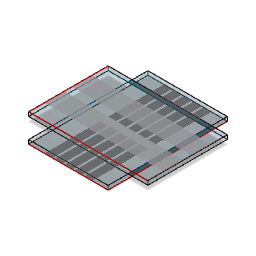
Assembly (Autodesk Fusion 360 archive; units mm, degrees)
design "TCA Test Structure"
Autodesk Fusion 360 part; units mm, degrees
sketch "Sketch1" plane through (0, 0, 0) normal (0, 1, 0) x (1, 0, 0)
  line L0 (10, -15) -> (-10, -15)
  line L1 (-10, -15) -> (-10, 15)
  line L2 (-10, 15) -> (10, 15)
  line L3 (10, 15) -> (10, -15)
  line L4 (10, -15) -> (-10, 15) construction
  line L5 (-10, -15) -> (10, 15) construction
  dimension "d1" = 20
  dimension "d2" = 30
  constraint perpendicular L0 L1
  constraint parallel L0 L2
  constraint parallel L1 L3
  constraint horizontal L0
  constraint coincident L4 origin
  constraint coincident L5 origin
  measures "d1" distance of L1.end L2.end
  measures "d2" distance of L0.end L1.end
extrude "Extrude1" add sketch "Sketch1" along normal blind 1
sketch "Sketch2" plane through (0, 1, 0) normal (0, 1, 0) x (-1, 0, 0)
  line L0 (-10, -15) -> (10, -15)
  line L1 (10, -15) -> (10, 15)
  line L2 (10, 15) -> (-10, 15)
  line L3 (-10, 15) -> (-10, -15)
  line L4 (-10, 10) -> (10, 10)
  line L5 (10, 10) -> (10, -10)
  line L6 (10, -10) -> (-10, -10)
  line L7 (-10, -10) -> (-10, 10)
  line L8 (-10, 10) -> (10, -10) construction
  line L9 (10, 10) -> (-10, -10) construction
  dimension "d5" = 20
  constraint perpendicular L4 L5
  constraint parallel L4 L6
  constraint parallel L5 L7
  constraint horizontal L4
  constraint coincident L3 L4.start
  constraint coincident L8 origin
  constraint coincident L9 origin
  measures "d5" distance of L4.end L5.end
extrude "Extrude2" add sketch "Sketch2" along normal blind 0.04 contours L1 L3 L4 L5 L6 L7
sketch "Sketch3" plane through (0, 1.04, 0) normal (0, 1, 0) x (-1, 0, 0)
  line L0 (-10, -10) -> (10, -10)
  line L1 (10, -10) -> (10, 10)
  line L2 (10, 10) -> (-10, 10)
  line L3 (-10, 10) -> (-10, -10)
  line L4 (-15, 10) -> (15, 10)
  line L5 (15, 10) -> (15, -10)
  line L6 (15, -10) -> (-15, -10)
  line L7 (-15, -10) -> (-15, 10)
  line L8 (-15, 10) -> (15, -10) construction
  line L9 (15, 10) -> (-15, -10) construction
  dimension "d8" = 30
  dimension "d9" = 20
  constraint perpendicular L4 L5
  constraint parallel L4 L6
  constraint parallel L5 L7
  constraint horizontal L4
  constraint coincident L8 origin
  constraint coincident L9 origin
  measures "d8" distance of L5.end L6.end
  measures "d9" distance of L4.end L5.end
extrude "Extrude3" add sketch "Sketch3" along normal blind 1

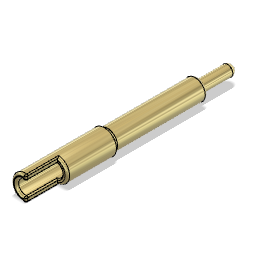
design "Pin-0955-0-15-20-71-14-11-0"
Autodesk Fusion 360 part; units mm, degrees
sketch "Sketch1" plane through (0, 0, 0) normal (0, 1, 0) x (1, 0, 0)
  line L0 (0, 0) -> (0, -7.65)
  line L1 (-0.445, 0) -> (0.445, 0)
  line L2 (0.445, 0) -> (0.445, -4.09)
  line L3 (0.445, -4.09) -> (-0.445, -4.09)
  line L4 (-0.445, -4.09) -> (-0.445, 0)
  line L5 (-0.535, -4.09) -> (0.535, -4.09)
  line L6 (0.535, -4.09) -> (0.535, -7.65)
  line L7 (0.535, -7.65) -> (-0.535, -7.65)
  line L8 (-0.535, -7.65) -> (-0.535, -4.09)
  line L9 (-0.305, -7.65) -> (0.305, -7.65)
  line L10 (0.305, -7.65) -> (0.305, -5.11)
  line L11 (0.305, -5.11) -> (-0.305, -5.11)
  line L12 (-0.305, -5.11) -> (-0.305, -7.65)
  line L13 (-0.24, 0) -> (0.24, 0)
  line L14 (0.24, 0) -> (0.24, 1.55)
  line L15 (0.24, 1.55) -> (-0.24, 1.55)
  line L16 (-0.24, 1.55) -> (-0.24, 0)
  circle A0 centre (-0.000074, 1.309926) radius 0.240074
  line L17 (0, 0) -> (0, 1.55)
  dimension "d1" = 7.65
  dimension "d2" = 4.09
  dimension "d3" = 0.89
  dimension "d4" = 3.56
  dimension "d5" = 1.07
  dimension "d6" = 0.61
  dimension "d7" = 2.54
  dimension "d8" = 0.48
  dimension "d9" = 1.55
  constraint coincident L0.start L17.start
  constraint vertical L0
  constraint horizontal L1
  constraint vertical L2
  constraint horizontal L3
  constraint vertical L4
  constraint midpoint L0.start L1
  constraint horizontal L5
  constraint vertical L6
  constraint horizontal L7
  constraint vertical L8
  constraint midpoint L0.end L7
  constraint horizontal L9
  constraint vertical L10
  constraint horizontal L11
  constraint vertical L12
  constraint midpoint L0.end L9
  constraint horizontal L13
  constraint vertical L14
  constraint horizontal L15
  constraint vertical L16
  constraint midpoint L0.start L13
  constraint tangent L14 A0
  constraint midpoint L15 L17.end
  measures "d1" distance of L0.start L0.end
  measures "d2" distance of L1.start L3.end
  measures "d3" distance of L1.start L1.end
  measures "d4" distance of L5.start L7.end
  measures "d5" distance of L6.end L7.end
  measures "d6" distance of L9.start L9.end
  measures "d7" distance of L9.start L11.end
  measures "d8" distance of L13.start L13.end
  measures "d9" distance of L13.start L15.end
revolve "Revolve1" add sketch "Sketch1" angle 360 about axis through (0, 0, 0) along (0, 0, 1) contours L0 L1 L3 L4 L5 L13 | L1 L13 L16 A0 L17 | L0 L3 L5 L7 L8 L11 L12 | A0 L17 picked at (-0.228333, -2.726667) picked at (-0.091391, 0.357428) picked at (-0.25, -4.43) picked at (-0.085672, 1.256662)
ref_plane "WorkPlane1" through (0.535, 0, 7.249122) normal (1, 0, 0) x (0, 1, 0)
sketch "Sketch3" plane through (0.535, 0, 7.249122) normal (1, 0, 0) x (0, 0, -1)
  line L0 (-0.400878, -0.7) -> (0.999122, -0.7)
  line L1 (0.999122, -0.7) -> (0.999122, 0.7)
  line L2 (0.999122, 0.7) -> (-0.400878, 0.7)
  line L3 (-0.400878, 0.7) -> (-0.400878, -0.7)
  line L4 (-0.400878, -0.7) -> (0.999122, 0.7) construction
  line L5 (0.999122, -0.7) -> (-0.400878, 0.7) construction
  point P0 (0.299122, 0)
  point P1 (-0.400878, 0)
  dimension "d18" = 1.4
  constraint horizontal L0
  constraint perpendicular L0 L1
  constraint parallel L0 L2
  constraint parallel L1 L3
extrude "Extrude2" cut sketch "Sketch3" against normal blind 0.435 contours L0 L1 L2 L3 picked at (0.065788, 0.233333)
fillet "Fillet1" radius 0.15 1 edges at (-0.414886, 0.160919, 4.09)
fillet "Fillet2" radius 0.1 6 edges at (0.535, 0, 6.25) (-0.414886, 0.160919, 0) (-0.535, 0, 7.65) (0.1, 0.406856, 7.65) (0.1, -0.406856, 7.65) (-0.305, 0, 7.65)
fillet "Fillet3" radius 0.05 9 edges at (0.065071, 0.495818, 7.625934) (0.1, 0.525571, 6.85) (0.1, 0.288141, 6.9) (0.068195, 0.329828, 7.62314) (0.068195, -0.329828, 7.62314) (0.1, -0.288141, 6.9) (0.1, -0.525571, 6.85) (0.065071, -0.495818, 7.625934) (0.305, 0, 6.25)
equation "d2 = 7.65 mm - 3.56 mm"
equation "d19 = ( -1.07 / 2 ) * 1 mm + 0.1 mm"
